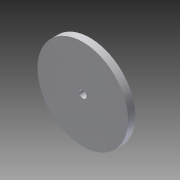
# Autodesk Inventor part: TapaFrontal
Saved by Autodesk Inventor 2013 (Build 170138000, 138)
## iProperties
Created: 2013-06-25
Part Number: TapaFrontal
Material: Genérico
Document SubType Name: Modeling
Designer: usuario
Density: 1 g/cm^3
Author: usuario
Autodesk Inventor part; units mm, degrees
ref_plane "YZ Plane" through (0, 0, 0) normal (1, 0, 0) x (0, 1, 0)
ref_plane "XZ Plane" through (0, 0, 0) normal (0, 1, 0) x (-1, 0, 0)
ref_plane "XY Plane" through (0, 0, 0) normal (0, 0, 1) x (1, 0, 0)
sketch "Boceto1" plane through (0, 0, 0) normal (0, 1, 0) x (-1, 0, 0)
  circle A0 centre (0, 0) radius 12.51
  dimension "d0" = 25.02
  constraints: 1 centre point, 1 coincident
  measures "d0" diameter of A0
extrude "Extrusión1" add sketch "Boceto1" along normal blind 2
sketch "Boceto2" plane through (0, 2, 0) normal (0, 1, 0) x (1, 0, 0)
  circle A0 centre (0, 0) radius 12.51 projected
  circle A1 centre (0, 0) radius 3.905
  dimension "d3" = 7.81
  constraints: 1 centre point, 1 coincident
  measures "d3" diameter of A1
extrude "Extrusión2" add sketch "Boceto2" along normal blind 2 contours A1
hole "Hole1" at (0, 4, 0) direction (0, -1, 0) diameter 5.2 depth 2
hole "Hole2" at (0, 2, 0) direction (0, -1, 0) diameter 2.02 end through all
